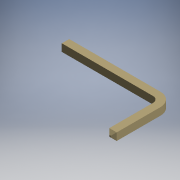
# Autodesk Inventor part: BF021-06-A-B-0400-0280-N-G_P
Saved by Autodesk Inventor 2017.3 (Build 213256000, 256)
## iProperties
Part Number: BF021-06-A-B-0400-0280-N-G_P
Material: Generic
Catalog Web Link: www.cadenas.de
Description: BF021 Pin-Header
Vendor: GCT
Document SubType Name: Modeling
Designer: partserver
Manufacturer: GCT
Mass: 0.00257159 g
Surface Area: 0.209409 cm^2
Volume: 0.00257159 cm^3
Density: 1 g/cm^3
Appearance: PSOLRGB-175-175-175
Category: PARTsolutions
Company: GCT
Title: BF021-06-A-B-0400-0280-N-G_P
Author: Cadenas PARTsolutions
Comments: Header
PSOL_IDENT_0: {$CADENAS_DATA\23d-libs\gct\b_t_b_connector\2_00mm\header\bf021\parts\bf021_header_pin.prj},224 {VTY
PSOL_IDENT_1: P=3D},{NB=BF021-06-A-B-0400-0280-N-G_P},{LINA=BF021-06-A-B-0400-0280-N-G_P},{NN=BF021 Pin},{DATE=06.
PSOL_IDENT_2: 12.2019 14:21:41},{GEOMDATE=22.02.2019 12:01:00},{VERSION=},{LINEID=10},{WBVAR=NOC,CP,W,C,D,IM,PO},{
PSOL_IDENT_3: WBNUMERIC=NOC,C,D}  {NB=BF021-06-A-B-0400-0280-N-G_P},{LINA=BF021-06-A-B-0400-0280-N-G_P},{KT=DUMMY}
PSOL_IDENT_4: ,{OC=BF021-06-A-B-0400-0280-N-G},{OCX=BF021},{NOC=6},{NOCX=6},{NOCXX=0},{CP=A},{W=B},{C=4.00},{CX=4.
PSOL_IDENT_5: 00,[1.00:10.00]},{CCX1=400},{CEXX=0},{D=2.80},{DDX=2.80,[1:6]},{DEXX=0},{DEX1=280},{IM=N},{PO=G},{PO
PSOL_IDENT_6: X= 'G', 'G = Plastic Box (Standard)','D', 'D = Tube', 'E'  , 'E = Tube with Cap'},{A=10.00},{B=12.00
PSOL_IDENT_7: },{OL=8.80},{WX=2.000},{COLR=0.784},{COLG=0.714},{COLB=0.529},{COLR2=0.784},{COLG2=0.714},{COLB2=0.5
PSOL_IDENT_8: 29},{DISCLAIMER=The creation and usage of 3D models generated by this builder are covered in our dis
PSOL_IDENT_9: claimer which can be viewed here}
NB: BF021-06-A-B-0400-0280-N-G_P
NN: BF021 Pin
NT: Header
NBSYN: $OC._P
LINA: BF021-06-A-B-0400-0280-N-G_P
CATALOG: Global Connector Technology
OC: BF021-06-A-B-0400-0280-N-G
NOC: 6
CP: A = Gold Flash All Over (Standard)
W: B = 2.00mm (Standard)
C: 4
D: 2.8
IM: N = Nylon 6T (Standard)
PO: G = Plastic Box (Standard)
A: 10
B: 12
DISCLAIMER: The creation and usage of 3D models generated by this builder are covered in our disclaimer which can be viewed here
SUPPLIER: GCT
ARTICLENO: BF021-06-A-B-0400-0280-N-G_P
BOMINFO: BF021-06-A-B-0400-0280-N-G_P
CREATOR: CADENAS GmbH
Autodesk Inventor part; units mm, degrees
sketch "Sketch_2" plane through (0, 0, 0) normal (0, 0, 1) x (1, 0, 0)
  line L0 (-0.5, -0.25) -> (3.8, -0.25)
  line L1 (3.8, -0.25) -> (4, -0.05)
  line L2 (4, -0.05) -> (4, 0.05)
  line L3 (4, 0.05) -> (3.8, 0.25)
  line L4 (3.8, 0.25) -> (-0.5, 0.25)
  line L5 (-0.5, 0.25) -> (-0.5, -0.25)
  constraints: 12 end point
extrude "Extrusion1" add sketch "Sketch_2" along normal mid plane 0.5
sketch "Sketch_3" plane through (0, 0, 0) normal (0, 0, 1) x (1, 0, 0)
  line L0 (-3.25, -3.6) -> (-3.05, -3.8)
  line L1 (-3.05, -3.8) -> (-2.95, -3.8)
  line L2 (-2.95, -3.8) -> (-2.75, -3.6)
  line L3 (-2.75, -3.6) -> (-2.75, -0.65)
  arc A0 (-2.35, -0.25) -> (-2.75, -0.65) centre (-2.35, -0.65) ccw
  line L4 (-2.35, -0.25) -> (-0.5, -0.25)
  line L5 (-0.5, -0.25) -> (-0.5, 0.25)
  line L6 (-0.5, 0.25) -> (-2.35, 0.25)
  arc A1 (-2.35, 0.25) -> (-3.25, -0.65) centre (-2.35, -0.65) ccw
  line L7 (-3.25, -0.65) -> (-3.25, -3.6)
  constraints: 16 end point, 4 point on circle, 2 centre point
extrude "Extrusion2" add sketch "Sketch_3" along normal mid plane 0.5
sketch "Sketch_4" plane through (0, 0, 0) normal (0, 1, 0) x (-1, 0, 0)
  line L0 (-3.7, -1.25) -> (-3.7, -0.25)
  line L1 (-3.7, -0.25) -> (-3.8, -0.25)
  line L2 (-3.8, -0.25) -> (-4, -0.05)
  line L3 (-4, -0.05) -> (-4, 0.05)
  line L4 (-4, 0.05) -> (-3.8, 0.25)
  line L5 (-3.8, 0.25) -> (-3.7, 0.25)
  line L6 (-3.7, 0.25) -> (-3.7, 1.25)
  line L7 (-3.7, 1.25) -> (-5, 1.25)
  line L8 (-5, 1.25) -> (-5, -1.25)
  line L9 (-5, -1.25) -> (-3.7, -1.25)
  constraints: 20 end point
extrude "Extrusion3" cut sketch "Sketch_4" along normal mid plane 0.5
sketch "Sketch_5" plane through (0, 0, 0) normal (1, 0, 0) x (0, 1, 0)
  line L0 (-4, 0.45) -> (-4, -0.45)
  line L1 (-4, -0.45) -> (-3.5, -0.45)
  line L2 (-3.5, -0.45) -> (-3.5, -0.25)
  line L3 (-3.5, -0.25) -> (-3.6, -0.25)
  line L4 (-3.6, -0.25) -> (-3.8, -0.05)
  line L5 (-3.8, -0.05) -> (-3.8, 0.05)
  line L6 (-3.8, 0.05) -> (-3.6, 0.25)
  line L7 (-3.6, 0.25) -> (-3.5, 0.25)
  line L8 (-3.5, 0.25) -> (-3.5, 0.45)
  line L9 (-3.5, 0.45) -> (-4, 0.45)
  constraints: 20 end point
extrude "Extrusion4" cut sketch "Sketch_5" against normal blind 3.5
ref_plane "IP_PIN_XY" through (0, 0, 0) normal (1, 0, 0) x (0, 0, -1)
ref_plane "IP_PIN_YZ" through (0, 0, 0) normal (0, 0, -1) x (0, 1, 0)
ref_plane "IP_PIN_ZX" through (0, 0, 0) normal (0, 1, 0) x (1, 0, 0)
body "Solid1"
